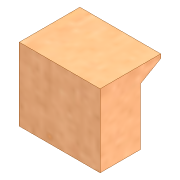
# Autodesk Inventor part: TNS-3-cover
Saved by Autodesk Inventor 2020 (Build 240168000, 168)
## iProperties
Created: 2021-06-28
Part Number: TNS-3-cover
Material: Generic
Document SubType Name: Modeling
Designer: Aidan Lee
Density: 1 g/cm^3
Appearance: Cherry - Natural Low Gloss
Author: Aidan Lee
Autodesk Inventor part; units mm, degrees
ref_plane "YZ Plane" through (0, 0, 0) normal (1, 0, 0) x (0, 1, 0)
ref_plane "XZ Plane" through (0, 0, 0) normal (0, 1, 0) x (-1, 0, 0)
ref_plane "XY Plane" through (0, 0, 0) normal (0, 0, 1) x (1, 0, 0)
sketch "Sketch1" plane through (0, 0, 0) normal (0, 0, 1) x (1, 0, 0)
  line L0 (0, 0) -> (20, 0)
  line L1 (20, 0) -> (20, 18)
  line L2 (20, 18) -> (0, 18)
  line L3 (0, 18) -> (0, 0)
  dimension "d0" = 20
  dimension "d1" = 18
  constraints: 8 end point, 2 parallel, 1 horizontal, 1 perpendicular
  measures "d0" distance of L0.start L0.end
  measures "d1" distance of L2.end L0.start
extrude "Extrusion1" add sketch "Sketch1" along normal blind 10
sketch "Sketch2" plane through (20, 0, 0) normal (1, 0, 0) x (0, 0, -1)
  line L0 (0, 0) -> (0, 18) projected
  line L1 (0, 18) -> (5, 18)
  line L2 (5, 18) -> (5, 17)
  line L3 (5, 17) -> (0, 14.1132)
  dimension "d4" = 5
  dimension "d5" = 60
  dimension "d6" = 1
  constraints: 6 end point, 1 horizontal, 1 point on line, 1 vertical
  measures "d4" distance of L0.end L1.end
  measures "d5" angle of L0 L3
  measures "d6" distance of L1.end L2.end
extrude "Extrusion2" add sketch "Sketch2" against normal up to surface (20 mm away)
body "Solid1"
